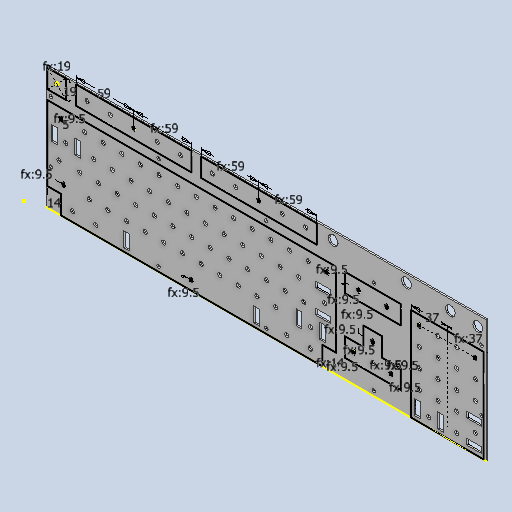
# Autodesk Inventor part: PCB
Saved by Autodesk Inventor 2025 (Build 290162000, 162)
## iProperties
Created: 2024-07-10
Part Number: PCB
Material: Generic
Document SubType Name: Modeling
Designer: adam
Density: 1 g/cm^3
Appearance: Default
Author: adam
Autodesk Inventor part; units mm, degrees
(part 1 of 2)
ref_plane "YZ Plane" through (0, 0, 0) normal (1, 0, 0) x (0, 1, 0)
ref_plane "XZ Plane" through (0, 0, 0) normal (0, 1, 0) x (-1, 0, 0)
ref_plane "XY Plane" through (0, 0, 0) normal (0, 0, 1) x (1, 0, 0)
sketch "Sketch2" plane through (0, 0, 0) normal (0, 0, 1) x (1, 0, 0)
  line L0 (313.1708, 72.3776) -> (298.1708, 72.3776) projected
  spline S0 degree 3 poles (439.2443, 124.4635) (438.3067, 125.4012) (437.0349, 125.928) (435.7088, 125.928) knots 0 0 0 0 1 1 1 1 projected
  line L1 (440.5, 108.25) -> (413, 108.25) projected
  spline S1 degree 3 poles (431.0894, 122.8414) (430.3155, 120.973) (430.7433, 118.8225) (432.1733, 117.3925) knots 0 0 0 0 1 1 1 1 projected
  spline S2 degree 3 poles (432.1733, 117.3925) (433.6033, 115.9625) (435.7538, 115.5347) (437.6222, 116.3086) knots 0 0 0 0 1 1 1 1 projected
  spline S3 degree 3 poles (435.7088, 125.928) (433.6865, 125.928) (431.8633, 124.7098) (431.0894, 122.8414) knots 0 0 0 0 1 1 1 1 projected
  line L2 (413, 115.25) -> (413, 127.25) projected
  line L3 (422.7108, 9.978) -> (422.7108, 24.978) projected
  line L4 (428.7108, 9.978) -> (422.7108, 9.978) projected
  line L5 (428.7108, 24.978) -> (428.7108, 9.978) projected
  line L6 (422.7108, 24.978) -> (428.7108, 24.978) projected
  line L7 (398.7108, 9.978) -> (398.7108, 24.978) projected
  line L8 (404.7108, 9.978) -> (398.7108, 9.978) projected
  line L9 (404.7108, 24.978) -> (404.7108, 9.978) projected
  line L10 (398.7108, 24.978) -> (404.7108, 24.978) projected
  line L11 (452.2088, 40.476) -> (452.2088, 34.476) projected
  spline S4 degree 3 poles (465.8832, 44.9197) (465.6123, 44.2658) (465.7621, 43.5131) (466.2626, 43.0126) knots 0 0 0 0 1 1 1 1 projected
  spline S5 degree 3 poles (467.5, 46) (466.7922, 46) (466.1541, 45.5736) (465.8832, 44.9197) knots 0 0 0 0 1 1 1 1 projected
  spline S6 degree 3 poles (466.2626, 43.0126) (466.7631, 42.5121) (467.5158, 42.3623) (468.1697, 42.6332) knots 0 0 0 0 1 1 1 1 projected
  spline S7 degree 3 poles (468.7374, 45.4874) (468.4092, 45.8156) (467.9641, 46) (467.5, 46) knots 0 0 0 0 1 1 1 1 projected
  spline S8 degree 3 poles (469.25, 44.25) (469.25, 44.7141) (469.0656, 45.1592) (468.7374, 45.4874) knots 0 0 0 0 1 1 1 1 projected
  spline S9 degree 3 poles (468.1697, 42.6332) (468.8236, 42.9041) (469.25, 43.5422) (469.25, 44.25) knots 0 0 0 0 1 1 1 1 projected
  spline S10 degree 3 poles (295.0681, 34.9296) (295.0681, 35.4922) (294.8446, 36.0318) (294.4468, 36.4296) knots 0 0 0 0 1 1 1 1 projected
  spline S11 degree 3 poles (358.7374, 107.6258) (358.4092, 107.954) (357.9641, 108.1384) (357.5, 108.1384) knots 0 0 0 0 1 1 1 1 projected
  spline S12 degree 3 poles (355.8832, 107.0581) (355.6123, 106.4042) (355.7621, 105.6515) (356.2626, 105.151) knots 0 0 0 0 1 1 1 1 projected
  spline S13 degree 3 poles (357.5, 108.1384) (356.7922, 108.1384) (356.1541, 107.712) (355.8832, 107.0581) knots 0 0 0 0 1 1 1 1 projected
  spline S14 degree 3 poles (356.2626, 105.151) (356.7631, 104.6505) (357.5158, 104.5007) (358.1697, 104.7716) knots 0 0 0 0 1 1 1 1 projected
  spline S15 degree 3 poles (358.1697, 104.7716) (358.8236, 105.0425) (359.25, 105.6806) (359.25, 106.3884) knots 0 0 0 0 1 1 1 1 projected
  line L12 (464, 108.25) -> (444.5, 108.25) projected
  spline S16 degree 3 poles (359.25, 106.3884) (359.25, 106.8525) (359.0656, 107.2976) (358.7374, 107.6258) knots 0 0 0 0 1 1 1 1 projected
  spline S17 degree 3 poles (440.7088, 120.928) (440.7088, 122.2541) (440.182, 123.5259) (439.2443, 124.4635) knots 0 0 0 0 1 1 1 1 projected
  spline S18 degree 3 poles (437.6222, 116.3086) (439.4906, 117.0825) (440.7088, 118.9057) (440.7088, 120.928) knots 0 0 0 0 1 1 1 1 projected
  spline S19 degree 3 poles (394.4023, 126.7719) (393.4647, 127.7096) (392.1929, 128.2364) (390.8668, 128.2364) knots 0 0 0 0 1 1 1 1 projected
  spline S20 degree 3 poles (395.8668, 123.2364) (395.8668, 124.5625) (395.34, 125.8343) (394.4023, 126.7719) knots 0 0 0 0 1 1 1 1 projected
  spline S21 degree 3 poles (392.7802, 118.617) (394.6486, 119.3909) (395.8668, 121.2141) (395.8668, 123.2364) knots 0 0 0 0 1 1 1 1 projected
  spline S22 degree 3 poles (387.3313, 119.7009) (388.7613, 118.2709) (390.9118, 117.8431) (392.7802, 118.617) knots 0 0 0 0 1 1 1 1 projected
  spline S23 degree 3 poles (386.2474, 125.1498) (385.4735, 123.2814) (385.9013, 121.1309) (387.3313, 119.7009) knots 0 0 0 0 1 1 1 1 projected
  spline S24 degree 3 poles (390.8668, 128.2364) (388.8445, 128.2364) (387.0213, 127.0182) (386.2474, 125.1498) knots 0 0 0 0 1 1 1 1 projected
  spline S25 degree 3 poles (465.8832, 107.0581) (465.6123, 106.4042) (465.7621, 105.6515) (466.2626, 105.151) knots 0 0 0 0 1 1 1 1 projected
  spline S26 degree 3 poles (466.2626, 105.151) (466.7631, 104.6505) (467.5158, 104.5007) (468.1697, 104.7716) knots 0 0 0 0 1 1 1 1 projected
  spline S27 degree 3 poles (467.5, 108.1384) (466.7922, 108.1384) (466.1541, 107.712) (465.8832, 107.0581) knots 0 0 0 0 1 1 1 1 projected
  spline S28 degree 3 poles (468.1697, 104.7716) (468.8236, 105.0425) (469.25, 105.6806) (469.25, 106.3884) knots 0 0 0 0 1 1 1 1 projected
  spline S29 degree 3 poles (468.7374, 107.6258) (468.4092, 107.954) (467.9641, 108.1384) (467.5, 108.1384) knots 0 0 0 0 1 1 1 1 projected
  spline S30 degree 3 poles (469.25, 106.3884) (469.25, 106.8525) (469.0656, 107.2976) (468.7374, 107.6258) knots 0 0 0 0 1 1 1 1 projected
  line L13 (413, 108.25) -> (413, 111.25) projected
  line L14 (452.2088, 16.476) -> (452.2088, 10.476) projected
  line L15 (467.2088, 16.476) -> (452.2088, 16.476) projected
  line L16 (467.2088, 10.476) -> (467.2088, 16.476) projected
  line L17 (452.2088, 10.476) -> (467.2088, 10.476) projected
  spline S31 degree 3 poles (467.2443, 124.4635) (466.3067, 125.4012) (465.0349, 125.928) (463.7088, 125.928) knots 0 0 0 0 1 1 1 1 projected
  line L18 (472.5, 131.25) -> (472.5, 6.25) projected
  spline S32 degree 3 poles (459.0894, 122.8414) (458.3155, 120.973) (458.7433, 118.8225) (460.1733, 117.3925) knots 0 0 0 0 1 1 1 1 projected
  spline S33 degree 3 poles (460.1733, 117.3925) (461.6033, 115.9625) (463.7538, 115.5347) (465.6222, 116.3086) knots 0 0 0 0 1 1 1 1 projected
  spline S34 degree 3 poles (463.7088, 125.928) (461.6865, 125.928) (459.8633, 124.7098) (459.0894, 122.8414) knots 0 0 0 0 1 1 1 1 projected
  spline S35 degree 3 poles (465.6222, 116.3086) (467.4906, 117.0825) (468.7088, 118.9057) (468.7088, 120.928) knots 0 0 0 0 1 1 1 1 projected
  spline S36 degree 3 poles (468.7088, 120.928) (468.7088, 122.2541) (468.182, 123.5259) (467.2443, 124.4635) knots 0 0 0 0 1 1 1 1 projected
  spline S37 degree 3 poles (206.0548, 74.5296) (205.657, 74.9274) (205.1174, 75.1509) (204.5548, 75.1509) knots 0 0 0 0 1 1 1 1 projected
  spline S38 degree 3 poles (206.6761, 73.0296) (206.6761, 73.5922) (206.4526, 74.1318) (206.0548, 74.5296) knots 0 0 0 0 1 1 1 1 projected
  spline S39 degree 3 poles (205.3666, 71.0698) (206.1593, 71.3981) (206.6761, 72.1716) (206.6761, 73.0296) knots 0 0 0 0 1 1 1 1 projected
  spline S40 degree 3 poles (203.0548, 71.5296) (203.6615, 70.9229) (204.5739, 70.7414) (205.3666, 71.0698) knots 0 0 0 0 1 1 1 1 projected
  spline S41 degree 3 poles (202.595, 73.8414) (202.2666, 73.0487) (202.4481, 72.1363) (203.0548, 71.5296) knots 0 0 0 0 1 1 1 1 projected
  spline S42 degree 3 poles (204.5548, 75.1509) (203.6968, 75.1509) (202.9233, 74.6341) (202.595, 73.8414) knots 0 0 0 0 1 1 1 1 projected
  spline S43 degree 3 poles (167.9548, 74.5296) (167.557, 74.9274) (167.0174, 75.1509) (166.4548, 75.1509) knots 0 0 0 0 1 1 1 1 projected
  spline S44 degree 3 poles (168.5761, 73.0296) (168.5761, 73.5922) (168.3526, 74.1318) (167.9548, 74.5296) knots 0 0 0 0 1 1 1 1 projected
  spline S45 degree 3 poles (167.2666, 71.0698) (168.0593, 71.3981) (168.5761, 72.1716) (168.5761, 73.0296) knots 0 0 0 0 1 1 1 1 projected
  spline S46 degree 3 poles (164.9548, 71.5296) (165.5615, 70.9229) (166.4739, 70.7414) (167.2666, 71.0698) knots 0 0 0 0 1 1 1 1 projected
  spline S47 degree 3 poles (164.495, 73.8414) (164.1666, 73.0487) (164.3481, 72.1363) (164.9548, 71.5296) knots 0 0 0 0 1 1 1 1 projected
  spline S48 degree 3 poles (166.4548, 75.1509) (165.5968, 75.1509) (164.8233, 74.6341) (164.495, 73.8414) knots 0 0 0 0 1 1 1 1 projected
  spline S49 degree 3 poles (187.0048, 74.5296) (186.607, 74.9274) (186.0674, 75.1509) (185.5048, 75.1509) knots 0 0 0 0 1 1 1 1 projected
  spline S50 degree 3 poles (183.545, 73.8414) (183.2166, 73.0487) (183.3981, 72.1363) (184.0048, 71.5296) knots 0 0 0 0 1 1 1 1 projected
  spline S51 degree 3 poles (187.6261, 73.0296) (187.6261, 73.5922) (187.4026, 74.1318) (187.0048, 74.5296) knots 0 0 0 0 1 1 1 1 projected
  spline S52 degree 3 poles (184.0048, 71.5296) (184.6115, 70.9229) (185.5239, 70.7414) (186.3166, 71.0698) knots 0 0 0 0 1 1 1 1 projected
  spline S53 degree 3 poles (186.3166, 71.0698) (187.1093, 71.3981) (187.6261, 72.1716) (187.6261, 73.0296) knots 0 0 0 0 1 1 1 1 projected
  spline S54 degree 3 poles (185.5048, 75.1509) (184.6468, 75.1509) (183.8733, 74.6341) (183.545, 73.8414) knots 0 0 0 0 1 1 1 1 projected
  spline S55 degree 3 poles (172.2728, 17.3796) (171.875, 17.7774) (171.3354, 18.0009) (170.7728, 18.0009) knots 0 0 0 0 1 1 1 1 projected
  spline S56 degree 3 poles (172.8941, 15.8796) (172.8941, 16.4422) (172.6706, 16.9818) (172.2728, 17.3796) knots 0 0 0 0 1 1 1 1 projected
  spline S57 degree 3 poles (171.5846, 13.9198) (172.3773, 14.2481) (172.8941, 15.0216) (172.8941, 15.8796) knots 0 0 0 0 1 1 1 1 projected
  spline S58 degree 3 poles (169.2728, 14.3796) (169.8795, 13.7729) (170.7919, 13.5914) (171.5846, 13.9198) knots 0 0 0 0 1 1 1 1 projected
  spline S59 degree 3 poles (168.813, 16.6914) (168.4846, 15.8987) (168.6661, 14.9863) (169.2728, 14.3796) knots 0 0 0 0 1 1 1 1 projected
  spline S60 degree 3 poles (170.7728, 18.0009) (169.9148, 18.0009) (169.1413, 17.4841) (168.813, 16.6914) knots 0 0 0 0 1 1 1 1 projected
  spline S61 degree 3 poles (201.4828, 36.4296) (201.085, 36.8274) (200.5454, 37.0509) (199.9828, 37.0509) knots 0 0 0 0 1 1 1 1 projected
  spline S62 degree 3 poles (202.1041, 34.9296) (202.1041, 35.4922) (201.8806, 36.0318) (201.4828, 36.4296) knots 0 0 0 0 1 1 1 1 projected
  spline S63 degree 3 poles (200.7946, 32.9698) (201.5873, 33.2981) (202.1041, 34.0716) (202.1041, 34.9296) knots 0 0 0 0 1 1 1 1 projected
  spline S64 degree 3 poles (198.4828, 33.4296) (199.0895, 32.8229) (200.0019, 32.6414) (200.7946, 32.9698) knots 0 0 0 0 1 1 1 1 projected
  spline S65 degree 3 poles (198.023, 35.7414) (197.6946, 34.9487) (197.8761, 34.0363) (198.4828, 33.4296) knots 0 0 0 0 1 1 1 1 projected
  spline S66 degree 3 poles (199.9828, 37.0509) (199.1248, 37.0509) (198.3513, 36.5341) (198.023, 35.7414) knots 0 0 0 0 1 1 1 1 projected
  spline S67 degree 3 poles (169.321, 54.7914) (168.9926, 53.9987) (169.1741, 53.0863) (169.7808, 52.4796) knots 0 0 0 0 1 1 1 1 projected
  spline S68 degree 3 poles (171.2808, 56.1009) (170.4228, 56.1009) (169.6493, 55.5841) (169.321, 54.7914) knots 0 0 0 0 1 1 1 1 projected
  spline S69 degree 3 poles (169.7808, 52.4796) (170.3875, 51.8729) (171.2999, 51.6914) (172.0926, 52.0198) knots 0 0 0 0 1 1 1 1 projected
  spline S70 degree 3 poles (172.7808, 55.4796) (172.383, 55.8774) (171.8434, 56.1009) (171.2808, 56.1009) knots 0 0 0 0 1 1 1 1 projected
  spline S71 degree 3 poles (172.0926, 52.0198) (172.8853, 52.3481) (173.4021, 53.1216) (173.4021, 53.9796) knots 0 0 0 0 1 1 1 1 projected
  spline S72 degree 3 poles (178.973, 35.7414) (178.6446, 34.9487) (178.8261, 34.0363) (179.4328, 33.4296) knots 0 0 0 0 1 1 1 1 projected
  spline S73 degree 3 poles (180.9328, 37.0509) (180.0748, 37.0509) (179.3013, 36.5341) (178.973, 35.7414) knots 0 0 0 0 1 1 1 1 projected
  spline S74 degree 3 poles (179.4328, 33.4296) (180.0395, 32.8229) (180.9519, 32.6414) (181.7446, 32.9698) knots 0 0 0 0 1 1 1 1 projected
  spline S75 degree 3 poles (182.4328, 36.4296) (182.035, 36.8274) (181.4954, 37.0509) (180.9328, 37.0509) knots 0 0 0 0 1 1 1 1 projected
  spline S76 degree 3 poles (181.7446, 32.9698) (182.5373, 33.2981) (183.0541, 34.0716) (183.0541, 34.9296) knots 0 0 0 0 1 1 1 1 projected
  spline S77 degree 3 poles (183.0541, 34.9296) (183.0541, 35.4922) (182.8306, 36.0318) (182.4328, 36.4296) knots 0 0 0 0 1 1 1 1 projected
  spline S78 degree 3 poles (188.371, 54.7914) (188.0426, 53.9987) (188.2241, 53.0863) (188.8308, 52.4796) knots 0 0 0 0 1 1 1 1 projected
  spline S79 degree 3 poles (190.3308, 56.1009) (189.4728, 56.1009) (188.6993, 55.5841) (188.371, 54.7914) knots 0 0 0 0 1 1 1 1 projected
  spline S80 degree 3 poles (188.8308, 52.4796) (189.4375, 51.8729) (190.3499, 51.6914) (191.1426, 52.0198) knots 0 0 0 0 1 1 1 1 projected
  spline S81 degree 3 poles (191.8308, 55.4796) (191.433, 55.8774) (190.8934, 56.1009) (190.3308, 56.1009) knots 0 0 0 0 1 1 1 1 projected
  spline S82 degree 3 poles (191.1426, 52.0198) (191.9353, 52.3481) (192.4521, 53.1216) (192.4521, 53.9796) knots 0 0 0 0 1 1 1 1 projected
  spline S83 degree 3 poles (192.4521, 53.9796) (192.4521, 54.5422) (192.2286, 55.0818) (191.8308, 55.4796) knots 0 0 0 0 1 1 1 1 projected
  spline S84 degree 3 poles (173.4021, 53.9796) (173.4021, 54.5422) (173.1786, 55.0818) (172.7808, 55.4796) knots 0 0 0 0 1 1 1 1 projected
  spline S85 degree 3 poles (159.1781, 92.0796) (159.1781, 93.2512) (158.2284, 94.2009) (157.0568, 94.2009) knots 0 0 0 0 1 1 1 1 projected
  spline S86 degree 3 poles (157.8686, 90.1198) (158.6613, 90.4481) (159.1781, 91.2216) (159.1781, 92.0796) knots 0 0 0 0 1 1 1 1 projected
  spline S87 degree 3 poles (193.6568, 90.5796) (194.2635, 89.9729) (195.1759, 89.7914) (195.9686, 90.1198) knots 0 0 0 0 1 1 1 1 projected
  spline S88 degree 3 poles (174.6068, 90.5796) (175.2135, 89.9729) (176.1259, 89.7914) (176.9186, 90.1198) knots 0 0 0 0 1 1 1 1 projected
  spline S89 degree 3 poles (176.9186, 90.1198) (177.7113, 90.4481) (178.2281, 91.2216) (178.2281, 92.0796) knots 0 0 0 0 1 1 1 1 projected
  spline S90 degree 3 poles (193.197, 92.8914) (192.8686, 92.0987) (193.0501, 91.1863) (193.6568, 90.5796) knots 0 0 0 0 1 1 1 1 projected
  spline S91 degree 3 poles (195.9686, 90.1198) (196.7613, 90.4481) (197.2781, 91.2216) (197.2781, 92.0796) knots 0 0 0 0 1 1 1 1 projected
  spline S92 degree 3 poles (197.2781, 92.0796) (197.2781, 92.6422) (197.0546, 93.1818) (196.6568, 93.5796) knots 0 0 0 0 1 1 1 1 projected
  spline S93 degree 3 poles (196.6568, 93.5796) (196.259, 93.9774) (195.7194, 94.2009) (195.1568, 94.2009) knots 0 0 0 0 1 1 1 1 projected
  spline S94 degree 3 poles (178.2281, 92.0796) (178.2281, 92.6422) (178.0046, 93.1818) (177.6068, 93.5796) knots 0 0 0 0 1 1 1 1 projected
  spline S95 degree 3 poles (195.1568, 94.2009) (194.2988, 94.2009) (193.5253, 93.6841) (193.197, 92.8914) knots 0 0 0 0 1 1 1 1 projected
  spline S96 degree 3 poles (177.6068, 93.5796) (177.209, 93.9774) (176.6694, 94.2009) (176.1068, 94.2009) knots 0 0 0 0 1 1 1 1 projected
  spline S97 degree 3 poles (176.1068, 94.2009) (175.2488, 94.2009) (174.4753, 93.6841) (174.147, 92.8914) knots 0 0 0 0 1 1 1 1 projected
  spline S98 degree 3 poles (155.5568, 90.5796) (156.1635, 89.9729) (157.0759, 89.7914) (157.8686, 90.1198) knots 0 0 0 0 1 1 1 1 projected
  spline S99 degree 3 poles (155.097, 92.8914) (154.7686, 92.0987) (154.9501, 91.1863) (155.5568, 90.5796) knots 0 0 0 0 1 1 1 1 projected
  spline S100 degree 3 poles (157.0568, 94.2009) (156.1988, 94.2009) (155.4253, 93.6841) (155.097, 92.8914) knots 0 0 0 0 1 1 1 1 projected
  spline S101 degree 3 poles (190.8568, 119.2364) (191.4635, 118.6297) (192.3759, 118.4482) (193.1686, 118.7766) knots 0 0 0 0 1 1 1 1 projected
  spline S102 degree 3 poles (193.1686, 118.7766) (193.9613, 119.1049) (194.4781, 119.8784) (194.4781, 120.7364) knots 0 0 0 0 1 1 1 1 projected
  spline S103 degree 3 poles (190.397, 121.5482) (190.0686, 120.7555) (190.2501, 119.8431) (190.8568, 119.2364) knots 0 0 0 0 1 1 1 1 projected
  spline S104 degree 3 poles (194.4781, 120.7364) (194.4781, 121.299) (194.2546, 121.8386) (193.8568, 122.2364) knots 0 0 0 0 1 1 1 1 projected
  spline S105 degree 3 poles (193.8568, 122.2364) (193.459, 122.6342) (192.9194, 122.8577) (192.3568, 122.8577) knots 0 0 0 0 1 1 1 1 projected
  spline S106 degree 3 poles (192.3568, 122.8577) (191.4988, 122.8577) (190.7253, 122.3409) (190.397, 121.5482) knots 0 0 0 0 1 1 1 1 projected
  spline S107 degree 3 poles (158.3508, 119.2364) (158.9575, 118.6297) (159.8699, 118.4482) (160.6626, 118.7766) knots 0 0 0 0 1 1 1 1 projected
  spline S108 degree 3 poles (160.6626, 118.7766) (161.4553, 119.1049) (161.9721, 119.8784) (161.9721, 120.7364) knots 0 0 0 0 1 1 1 1 projected
  spline S109 degree 3 poles (161.9721, 120.7364) (161.9721, 121.299) (161.7486, 121.8386) (161.3508, 122.2364) knots 0 0 0 0 1 1 1 1 projected
  spline S110 degree 3 poles (157.891, 121.5482) (157.5626, 120.7555) (157.7441, 119.8431) (158.3508, 119.2364) knots 0 0 0 0 1 1 1 1 projected
  spline S111 degree 3 poles (161.3508, 122.2364) (160.953, 122.6342) (160.4134, 122.8577) (159.8508, 122.8577) knots 0 0 0 0 1 1 1 1 projected
  spline S112 degree 3 poles (159.8508, 122.8577) (158.9928, 122.8577) (158.2193, 122.3409) (157.891, 121.5482) knots 0 0 0 0 1 1 1 1 projected
  spline S113 degree 3 poles (174.147, 92.8914) (173.8186, 92.0987) (174.0001, 91.1863) (174.6068, 90.5796) knots 0 0 0 0 1 1 1 1 projected
  spline S114 degree 3 poles (164.0041, 34.9296) (164.0041, 36.1012) (163.0544, 37.0509) (161.8828, 37.0509) knots 0 0 0 0 1 1 1 1 projected
  spline S115 degree 3 poles (162.6946, 32.9698) (163.4873, 33.2981) (164.0041, 34.0716) (164.0041, 34.9296) knots 0 0 0 0 1 1 1 1 projected
  spline S116 degree 3 poles (160.3828, 33.4296) (160.9895, 32.8229) (161.9019, 32.6414) (162.6946, 32.9698) knots 0 0 0 0 1 1 1 1 projected
  spline S117 degree 3 poles (159.923, 35.7414) (159.5946, 34.9487) (159.7761, 34.0363) (160.3828, 33.4296) knots 0 0 0 0 1 1 1 1 projected
  spline S118 degree 3 poles (161.8828, 37.0509) (161.0248, 37.0509) (160.2513, 36.5341) (159.923, 35.7414) knots 0 0 0 0 1 1 1 1 projected
  spline S119 degree 3 poles (154.3521, 53.9796) (154.3521, 55.1512) (153.4024, 56.1009) (152.2308, 56.1009) knots 0 0 0 0 1 1 1 1 projected
  spline S120 degree 3 poles (153.0426, 52.0198) (153.8353, 52.3481) (154.3521, 53.1216) (154.3521, 53.9796) knots 0 0 0 0 1 1 1 1 projected
  spline S121 degree 3 poles (150.271, 54.7914) (149.9426, 53.9987) (150.1241, 53.0863) (150.7308, 52.4796) knots 0 0 0 0 1 1 1 1 projected
  spline S122 degree 3 poles (150.7308, 52.4796) (151.3375, 51.8729) (152.2499, 51.6914) (153.0426, 52.0198) knots 0 0 0 0 1 1 1 1 projected
  spline S123 degree 3 poles (152.2308, 56.1009) (151.3728, 56.1009) (150.5993, 55.5841) (150.271, 54.7914) knots 0 0 0 0 1 1 1 1 projected
  spline S124 degree 3 poles (139.25, 11.25) (139.25, 11.7141) (139.0656, 12.1592) (138.7374, 12.4874) knots 0 0 0 0 1 1 1 1 projected
  spline S125 degree 3 poles (138.7374, 12.4874) (138.4092, 12.8156) (137.9641, 13) (137.5, 13) knots 0 0 0 0 1 1 1 1 projected
  spline S126 degree 3 poles (138.1697, 9.6332) (138.8236, 9.9041) (139.25, 10.5422) (139.25, 11.25) knots 0 0 0 0 1 1 1 1 projected
  spline S127 degree 3 poles (137.5, 13) (136.7922, 13) (136.1541, 12.5736) (135.8832, 11.9197) knots 0 0 0 0 1 1 1 1 projected
  spline S128 degree 3 poles (135.8832, 11.9197) (135.6123, 11.2658) (135.7621, 10.5131) (136.2626, 10.0126) knots 0 0 0 0 1 1 1 1 projected
  spline S129 degree 3 poles (136.2626, 10.0126) (136.7631, 9.5121) (137.5158, 9.3623) (138.1697, 9.6332) knots 0 0 0 0 1 1 1 1 projected
  spline S130 degree 3 poles (148.9048, 74.4508) (148.507, 74.8486) (147.9674, 75.0721) (147.4048, 75.0721) knots 0 0 0 0 1 1 1 1 projected
  spline S131 degree 3 poles (149.5261, 72.9508) (149.5261, 73.5134) (149.3026, 74.053) (148.9048, 74.4508) knots 0 0 0 0 1 1 1 1 projected
  spline S132 degree 3 poles (120.4568, 93.5796) (120.059, 93.9774) (119.5194, 94.2009) (118.9568, 94.2009) knots 0 0 0 0 1 1 1 1 projected
  spline S133 degree 3 poles (118.9568, 94.2009) (117.7852, 94.2009) (116.8355, 93.2512) (116.8355, 92.0796) knots 0 0 0 0 1 1 1 1 projected
  spline S134 degree 3 poles (121.0781, 92.0796) (121.0781, 92.6422) (120.8546, 93.1818) (120.4568, 93.5796) knots 0 0 0 0 1 1 1 1 projected
  spline S135 degree 3 poles (116.8355, 92.0796) (116.8355, 90.908) (117.7852, 89.9583) (118.9568, 89.9583) knots 0 0 0 0 1 1 1 1 projected
  spline S136 degree 3 poles (118.9568, 89.9583) (120.1284, 89.9583) (121.0781, 90.908) (121.0781, 92.0796) knots 0 0 0 0 1 1 1 1 projected
  spline S137 degree 3 poles (138.0068, 94.2009) (137.1488, 94.2009) (136.3753, 93.6841) (136.047, 92.8914) knots 0 0 0 0 1 1 1 1 projected
  spline S138 degree 3 poles (139.5068, 93.5796) (139.109, 93.9774) (138.5694, 94.2009) (138.0068, 94.2009) knots 0 0 0 0 1 1 1 1 projected
  spline S139 degree 3 poles (140.1281, 92.0796) (140.1281, 92.6422) (139.9046, 93.1818) (139.5068, 93.5796) knots 0 0 0 0 1 1 1 1 projected
  spline S140 degree 3 poles (136.047, 92.8914) (135.7186, 92.0987) (135.9001, 91.1863) (136.5068, 90.5796) knots 0 0 0 0 1 1 1 1 projected
  spline S141 degree 3 poles (138.8186, 90.1198) (139.6113, 90.4481) (140.1281, 91.2216) (140.1281, 92.0796) knots 0 0 0 0 1 1 1 1 projected
  spline S142 degree 3 poles (129.8548, 74.5296) (129.457, 74.9274) (128.9174, 75.1509) (128.3548, 75.1509) knots 0 0 0 0 1 1 1 1 projected
  spline S143 degree 3 poles (147.4048, 75.0721) (146.5468, 75.0721) (145.7733, 74.5553) (145.445, 73.7626) knots 0 0 0 0 1 1 1 1 projected
  spline S144 degree 3 poles (145.445, 73.7626) (145.1166, 72.9699) (145.2981, 72.0575) (145.9048, 71.4508) knots 0 0 0 0 1 1 1 1 projected
  spline S145 degree 3 poles (148.2166, 70.991) (149.0093, 71.3193) (149.5261, 72.0928) (149.5261, 72.9508) knots 0 0 0 0 1 1 1 1 projected
  spline S146 degree 3 poles (145.9048, 71.4508) (146.5115, 70.8441) (147.4239, 70.6626) (148.2166, 70.991) knots 0 0 0 0 1 1 1 1 projected
  spline S147 degree 3 poles (128.3548, 75.1509) (127.4968, 75.1509) (126.7233, 74.6341) (126.395, 73.8414) knots 0 0 0 0 1 1 1 1 projected
  spline S148 degree 3 poles (130.4761, 73.0296) (130.4761, 73.5922) (130.2526, 74.1318) (129.8548, 74.5296) knots 0 0 0 0 1 1 1 1 projected
  spline S149 degree 3 poles (126.395, 73.8414) (126.0666, 73.0487) (126.2481, 72.1363) (126.8548, 71.5296) knots 0 0 0 0 1 1 1 1 projected
  spline S150 degree 3 poles (129.1666, 71.0698) (129.9593, 71.3981) (130.4761, 72.1716) (130.4761, 73.0296) knots 0 0 0 0 1 1 1 1 projected
  spline S151 degree 3 poles (126.8548, 71.5296) (127.4615, 70.9229) (128.3739, 70.7414) (129.1666, 71.0698) knots 0 0 0 0 1 1 1 1 projected
  spline S152 degree 3 poles (136.5068, 90.5796) (137.1135, 89.9729) (138.0259, 89.7914) (138.8186, 90.1198) knots 0 0 0 0 1 1 1 1 projected
  spline S153 degree 3 poles (138.7374, 107.6258) (138.4092, 107.954) (137.9641, 108.1384) (137.5, 108.1384) knots 0 0 0 0 1 1 1 1 projected
  spline S154 degree 3 poles (139.25, 106.3884) (139.25, 106.8525) (139.0656, 107.2976) (138.7374, 107.6258) knots 0 0 0 0 1 1 1 1 projected
  spline S155 degree 3 poles (138.1697, 104.7716) (138.8236, 105.0425) (139.25, 105.6806) (139.25, 106.3884) knots 0 0 0 0 1 1 1 1 projected
  spline S156 degree 3 poles (136.2626, 105.151) (136.7631, 104.6505) (137.5158, 104.5007) (138.1697, 104.7716) knots 0 0 0 0 1 1 1 1 projected
  spline S157 degree 3 poles (135.8832, 107.0581) (135.6123, 106.4042) (135.7621, 105.6515) (136.2626, 105.151) knots 0 0 0 0 1 1 1 1 projected
  spline S158 degree 3 poles (137.5, 108.1384) (136.7922, 108.1384) (136.1541, 107.712) (135.8832, 107.0581) knots 0 0 0 0 1 1 1 1 projected
  spline S159 degree 3 poles (134.4748, 119.2364) (135.0815, 118.6297) (135.9939, 118.4482) (136.7866, 118.7766) knots 0 0 0 0 1 1 1 1 projected
  spline S160 degree 3 poles (136.7866, 118.7766) (137.5793, 119.1049) (138.0961, 119.8784) (138.0961, 120.7364) knots 0 0 0 0 1 1 1 1 projected
  spline S161 degree 3 poles (134.015, 121.5482) (133.6866, 120.7555) (133.8681, 119.8431) (134.4748, 119.2364) knots 0 0 0 0 1 1 1 1 projected
  spline S162 degree 3 poles (137.4748, 122.2364) (137.077, 122.6342) (136.5374, 122.8577) (135.9748, 122.8577) knots 0 0 0 0 1 1 1 1 projected
  spline S163 degree 3 poles (135.9748, 122.8577) (135.1168, 122.8577) (134.3433, 122.3409) (134.015, 121.5482) knots 0 0 0 0 1 1 1 1 projected
  spline S164 degree 3 poles (112.9106, 118.7486) (113.7033, 119.0769) (114.2201, 119.8504) (114.2201, 120.7084) knots 0 0 0 0 1 1 1 1 projected
  spline S165 degree 3 poles (110.5988, 119.2084) (111.2055, 118.6017) (112.1179, 118.4202) (112.9106, 118.7486) knots 0 0 0 0 1 1 1 1 projected
  spline S166 degree 3 poles (114.2201, 120.7084) (114.2201, 121.271) (113.9966, 121.8106) (113.5988, 122.2084) knots 0 0 0 0 1 1 1 1 projected
  spline S167 degree 3 poles (113.5988, 122.2084) (113.201, 122.6062) (112.6614, 122.8297) (112.0988, 122.8297) knots 0 0 0 0 1 1 1 1 projected
  spline S168 degree 3 poles (110.139, 121.5202) (109.8106, 120.7275) (109.9921, 119.8151) (110.5988, 119.2084) knots 0 0 0 0 1 1 1 1 projected
  spline S169 degree 3 poles (112.0988, 122.8297) (111.2408, 122.8297) (110.4673, 122.3129) (110.139, 121.5202) knots 0 0 0 0 1 1 1 1 projected
  spline S170 degree 3 poles (138.0961, 120.7364) (138.0961, 121.299) (137.8726, 121.8386) (137.4748, 122.2364) knots 0 0 0 0 1 1 1 1 projected
  line L19 (101.6246, 24.8046) -> (107.6246, 24.8046) projected
  spline S171 degree 3 poles (135.3021, 53.9796) (135.3021, 54.5422) (135.0786, 55.0818) (134.6808, 55.4796) knots 0 0 0 0 1 1 1 1 projected
  spline S172 degree 3 poles (133.9926, 52.0198) (134.7853, 52.3481) (135.3021, 53.1216) (135.3021, 53.9796) knots 0 0 0 0 1 1 1 1 projected
  spline S173 degree 3 poles (134.6808, 55.4796) (134.283, 55.8774) (133.7434, 56.1009) (133.1808, 56.1009) knots 0 0 0 0 1 1 1 1 projected
  spline S174 degree 3 poles (131.6808, 52.4796) (132.2875, 51.8729) (133.1999, 51.6914) (133.9926, 52.0198) knots 0 0 0 0 1 1 1 1 projected
  spline S175 degree 3 poles (144.3328, 36.4296) (143.935, 36.8274) (143.3954, 37.0509) (142.8328, 37.0509) knots 0 0 0 0 1 1 1 1 projected
  spline S176 degree 3 poles (133.1808, 56.1009) (132.3228, 56.1009) (131.5493, 55.5841) (131.221, 54.7914) knots 0 0 0 0 1 1 1 1 projected
  spline S177 degree 3 poles (131.221, 54.7914) (130.8926, 53.9987) (131.0741, 53.0863) (131.6808, 52.4796) knots 0 0 0 0 1 1 1 1 projected
  spline S178 degree 3 poles (144.9541, 34.9296) (144.9541, 35.4922) (144.7306, 36.0318) (144.3328, 36.4296) knots 0 0 0 0 1 1 1 1 projected
  spline S179 degree 3 poles (142.8328, 37.0509) (141.9748, 37.0509) (141.2013, 36.5341) (140.873, 35.7414) knots 0 0 0 0 1 1 1 1 projected
  spline S180 degree 3 poles (140.873, 35.7414) (140.5446, 34.9487) (140.7261, 34.0363) (141.3328, 33.4296) knots 0 0 0 0 1 1 1 1 projected
  spline S181 degree 3 poles (141.3328, 33.4296) (141.9395, 32.8229) (142.8519, 32.6414) (143.6446, 32.9698) knots 0 0 0 0 1 1 1 1 projected
  spline S182 degree 3 poles (125.9041, 34.9296) (125.9041, 35.4922) (125.6806, 36.0318) (125.2828, 36.4296) knots 0 0 0 0 1 1 1 1 projected
  spline S183 degree 3 poles (125.2828, 36.4296) (124.885, 36.8274) (124.3454, 37.0509) (123.7828, 37.0509) knots 0 0 0 0 1 1 1 1 projected
  spline S184 degree 3 poles (116.2521, 53.9796) (116.2521, 54.5422) (116.0286, 55.0818) (115.6308, 55.4796) knots 0 0 0 0 1 1 1 1 projected
  spline S185 degree 3 poles (114.9426, 52.0198) (115.7353, 52.3481) (116.2521, 53.1216) (116.2521, 53.9796) knots 0 0 0 0 1 1 1 1 projected
  spline S186 degree 3 poles (115.6308, 55.4796) (115.233, 55.8774) (114.6934, 56.1009) (114.1308, 56.1009) knots 0 0 0 0 1 1 1 1 projected
  spline S187 degree 3 poles (114.1308, 56.1009) (113.2728, 56.1009) (112.4993, 55.5841) (112.171, 54.7914) knots 0 0 0 0 1 1 1 1 projected
  spline S188 degree 3 poles (112.171, 54.7914) (111.8426, 53.9987) (112.0241, 53.0863) (112.6308, 52.4796) knots 0 0 0 0 1 1 1 1 projected
  spline S189 degree 3 poles (112.6308, 52.4796) (113.2375, 51.8729) (114.1499, 51.6914) (114.9426, 52.0198) knots 0 0 0 0 1 1 1 1 projected
  spline S190 degree 3 poles (124.5946, 32.9698) (125.3873, 33.2981) (125.9041, 34.0716) (125.9041, 34.9296) knots 0 0 0 0 1 1 1 1 projected
  spline S191 degree 3 poles (123.7828, 37.0509) (122.9248, 37.0509) (122.1513, 36.5341) (121.823, 35.7414) knots 0 0 0 0 1 1 1 1 projected
  spline S192 degree 3 poles (122.2828, 33.4296) (122.8895, 32.8229) (123.8019, 32.6414) (124.5946, 32.9698) knots 0 0 0 0 1 1 1 1 projected
  spline S193 degree 3 poles (121.823, 35.7414) (121.4946, 34.9487) (121.6761, 34.0363) (122.2828, 33.4296) knots 0 0 0 0 1 1 1 1 projected
  spline S194 degree 3 poles (106.8541, 34.9296) (106.8541, 35.4922) (106.6306, 36.0318) (106.2328, 36.4296) knots 0 0 0 0 1 1 1 1 projected
  spline S195 degree 3 poles (106.2328, 36.4296) (105.835, 36.8274) (105.2954, 37.0509) (104.7328, 37.0509) knots 0 0 0 0 1 1 1 1 projected
  spline S196 degree 3 poles (105.5446, 32.9698) (106.3373, 33.2981) (106.8541, 34.0716) (106.8541, 34.9296) knots 0 0 0 0 1 1 1 1 projected
  spline S197 degree 3 poles (104.7328, 37.0509) (103.8748, 37.0509) (103.1013, 36.5341) (102.773, 35.7414) knots 0 0 0 0 1 1 1 1 projected
  spline S198 degree 3 poles (102.773, 35.7414) (102.4446, 34.9487) (102.6261, 34.0363) (103.2328, 33.4296) knots 0 0 0 0 1 1 1 1 projected
  spline S199 degree 3 poles (103.2328, 33.4296) (103.8395, 32.8229) (104.7519, 32.6414) (105.5446, 32.9698) knots 0 0 0 0 1 1 1 1 projected
  spline S200 degree 3 poles (143.6446, 32.9698) (144.4373, 33.2981) (144.9541, 34.0716) (144.9541, 34.9296) knots 0 0 0 0 1 1 1 1 projected
  spline S201 degree 3 poles (111.4261, 73.0296) (111.4261, 73.5922) (111.2026, 74.1318) (110.8048, 74.5296) knots 0 0 0 0 1 1 1 1 projected
  spline S202 degree 3 poles (110.8048, 74.5296) (110.407, 74.9274) (109.8674, 75.1509) (109.3048, 75.1509) knots 0 0 0 0 1 1 1 1 projected
  spline S203 degree 3 poles (110.1166, 71.0698) (110.9093, 71.3981) (111.4261, 72.1716) (111.4261, 73.0296) knots 0 0 0 0 1 1 1 1 projected
  spline S204 degree 3 poles (109.3048, 75.1509) (108.4468, 75.1509) (107.6733, 74.6341) (107.345, 73.8414) knots 0 0 0 0 1 1 1 1 projected
  spline S205 degree 3 poles (107.8048, 71.5296) (108.4115, 70.9229) (109.3239, 70.7414) (110.1166, 71.0698) knots 0 0 0 0 1 1 1 1 projected
  spline S206 degree 3 poles (107.345, 73.8414) (107.0166, 73.0487) (107.1981, 72.1363) (107.8048, 71.5296) knots 0 0 0 0 1 1 1 1 projected
  spline S207 degree 3 poles (102.0281, 92.0796) (102.0281, 92.6422) (101.8046, 93.1818) (101.4068, 93.5796) knots 0 0 0 0 1 1 1 1 projected
  spline S208 degree 3 poles (100.7186, 90.1198) (101.5113, 90.4481) (102.0281, 91.2216) (102.0281, 92.0796) knots 0 0 0 0 1 1 1 1 projected
  spline S209 degree 3 poles (101.4068, 93.5796) (101.009, 93.9774) (100.4694, 94.2009) (99.9068, 94.2009) knots 0 0 0 0 1 1 1 1 projected
  spline S210 degree 3 poles (99.9068, 94.2009) (99.0488, 94.2009) (98.2753, 93.6841) (97.947, 92.8914) knots 0 0 0 0 1 1 1 1 projected
  spline S211 degree 3 poles (98.4068, 90.5796) (99.0135, 89.9729) (99.9259, 89.7914) (100.7186, 90.1198) knots 0 0 0 0 1 1 1 1 projected
  spline S212 degree 3 poles (92.3761, 73.0296) (92.3761, 73.5922) (92.1526, 74.1318) (91.7548, 74.5296) knots 0 0 0 0 1 1 1 1 projected
  spline S213 degree 3 poles (91.7548, 74.5296) (91.357, 74.9274) (90.8174, 75.1509) (90.2548, 75.1509) knots 0 0 0 0 1 1 1 1 projected
  spline S214 degree 3 poles (91.0666, 71.0698) (91.8593, 71.3981) (92.3761, 72.1716) (92.3761, 73.0296) knots 0 0 0 0 1 1 1 1 projected
  spline S215 degree 3 poles (90.2548, 75.1509) (89.3968, 75.1509) (88.6233, 74.6341) (88.295, 73.8414) knots 0 0 0 0 1 1 1 1 projected
  spline S216 degree 3 poles (88.7548, 71.5296) (89.3615, 70.9229) (90.2739, 70.7414) (91.0666, 71.0698) knots 0 0 0 0 1 1 1 1 projected
  spline S217 degree 3 poles (88.295, 73.8414) (87.9666, 73.0487) (88.1481, 72.1363) (88.7548, 71.5296) knots 0 0 0 0 1 1 1 1 projected
  spline S218 degree 3 poles (97.947, 92.8914) (97.6186, 92.0987) (97.8001, 91.1863) (98.4068, 90.5796) knots 0 0 0 0 1 1 1 1 projected
  spline S219 degree 3 poles (89.0346, 118.7766) (89.8273, 119.1049) (90.3441, 119.8784) (90.3441, 120.7364) knots 0 0 0 0 1 1 1 1 projected
  spline S220 degree 3 poles (72.7048, 74.5296) (72.307, 74.9274) (71.7674, 75.1509) (71.2048, 75.1509) knots 0 0 0 0 1 1 1 1 projected
  spline S221 degree 3 poles (73.3261, 73.0296) (73.3261, 73.5922) (73.1026, 74.1318) (72.7048, 74.5296) knots 0 0 0 0 1 1 1 1 projected
  spline S222 degree 3 poles (72.0166, 71.0698) (72.8093, 71.3981) (73.3261, 72.1716) (73.3261, 73.0296) knots 0 0 0 0 1 1 1 1 projected
  spline S223 degree 3 poles (69.7048, 71.5296) (70.3115, 70.9229) (71.2239, 70.7414) (72.0166, 71.0698) knots 0 0 0 0 1 1 1 1 projected
  spline S224 degree 3 poles (69.245, 73.8414) (68.9166, 73.0487) (69.0981, 72.1363) (69.7048, 71.5296) knots 0 0 0 0 1 1 1 1 projected
  spline S225 degree 3 poles (71.2048, 75.1509) (70.3468, 75.1509) (69.5733, 74.6341) (69.245, 73.8414) knots 0 0 0 0 1 1 1 1 projected
  spline S226 degree 3 poles (60.3068, 90.5796) (60.9135, 89.9729) (61.8259, 89.7914) (62.6186, 90.1198) knots 0 0 0 0 1 1 1 1 projected
  spline S227 degree 3 poles (59.847, 92.8914) (59.5186, 92.0987) (59.7001, 91.1863) (60.3068, 90.5796) knots 0 0 0 0 1 1 1 1 projected
  spline S228 degree 3 poles (62.6186, 90.1198) (63.4113, 90.4481) (63.9281, 91.2216) (63.9281, 92.0796) knots 0 0 0 0 1 1 1 1 projected
  spline S229 degree 3 poles (63.9281, 92.0796) (63.9281, 92.6422) (63.7046, 93.1818) (63.3068, 93.5796) knots 0 0 0 0 1 1 1 1 projected
  spline S230 degree 3 poles (63.3068, 93.5796) (62.909, 93.9774) (62.3694, 94.2009) (61.8068, 94.2009) knots 0 0 0 0 1 1 1 1 projected
  spline S231 degree 3 poles (78.897, 92.8914) (78.5686, 92.0987) (78.7501, 91.1863) (79.3568, 90.5796) knots 0 0 0 0 1 1 1 1 projected
  spline S232 degree 3 poles (79.3568, 90.5796) (79.9635, 89.9729) (80.8759, 89.7914) (81.6686, 90.1198) knots 0 0 0 0 1 1 1 1 projected
  spline S233 degree 3 poles (80.8568, 94.2009) (79.9988, 94.2009) (79.2253, 93.6841) (78.897, 92.8914) knots 0 0 0 0 1 1 1 1 projected
  spline S234 degree 3 poles (81.6686, 90.1198) (82.4613, 90.4481) (82.9781, 91.2216) (82.9781, 92.0796) knots 0 0 0 0 1 1 1 1 projected
  spline S235 degree 3 poles (82.9781, 92.0796) (82.9781, 93.2512) (82.0284, 94.2009) (80.8568, 94.2009) knots 0 0 0 0 1 1 1 1 projected
  spline S236 degree 3 poles (61.8068, 94.2009) (60.9488, 94.2009) (60.1753, 93.6841) (59.847, 92.8914) knots 0 0 0 0 1 1 1 1 projected
  spline S237 degree 3 poles (50.1726, 13.9198) (50.9653, 14.2481) (51.4821, 15.0216) (51.4821, 15.8796) knots 0 0 0 0 1 1 1 1 projected
  spline S238 degree 3 poles (50.8608, 17.3796) (50.463, 17.7774) (49.9234, 18.0009) (49.3608, 18.0009) knots 0 0 0 0 1 1 1 1 projected
  spline S239 degree 3 poles (49.3608, 18.0009) (48.5028, 18.0009) (47.7293, 17.4841) (47.401, 16.6914) knots 0 0 0 0 1 1 1 1 projected
  spline S240 degree 3 poles (47.8608, 14.3796) (48.4675, 13.7729) (49.3799, 13.5914) (50.1726, 13.9198) knots 0 0 0 0 1 1 1 1 projected
  spline S241 degree 3 poles (47.401, 16.6914) (47.0726, 15.8987) (47.2541, 14.9863) (47.8608, 14.3796) knots 0 0 0 0 1 1 1 1 projected
  spline S242 degree 3 poles (51.4821, 15.8796) (51.4821, 16.4422) (51.2586, 16.9818) (50.8608, 17.3796) knots 0 0 0 0 1 1 1 1 projected
  line L20 (51.7568, 67.0296) -> (51.7568, 82.0296) projected
  line L21 (57.7568, 67.0296) -> (51.7568, 67.0296) projected
  line L22 (57.7568, 82.0296) -> (57.7568, 67.0296) projected
  line L23 (51.7568, 82.0296) -> (57.7568, 82.0296) projected
  line L24 (27.7568, 67.0296) -> (27.7568, 82.0296) projected
  line L25 (33.7568, 67.0296) -> (27.7568, 67.0296) projected
  line L26 (33.7568, 82.0296) -> (33.7568, 67.0296) projected
  line L27 (27.7568, 82.0296) -> (33.7568, 82.0296) projected
  spline S243 degree 3 poles (40.1501, 92.0796) (40.1501, 92.6422) (39.9266, 93.1818) (39.5288, 93.5796) knots 0 0 0 0 1 1 1 1 projected
  spline S244 degree 3 poles (39.5288, 93.5796) (39.131, 93.9774) (38.5914, 94.2009) (38.0288, 94.2009) knots 0 0 0 0 1 1 1 1 projected
  spline S245 degree 3 poles (38.0288, 89.9583) (39.2004, 89.9583) (40.1501, 90.908) (40.1501, 92.0796) knots 0 0 0 0 1 1 1 1 projected
  spline S246 degree 3 poles (38.0288, 94.2009) (36.8572, 94.2009) (35.9075, 93.2512) (35.9075, 92.0796) knots 0 0 0 0 1 1 1 1 projected
  spline S247 degree 3 poles (35.9075, 92.0796) (35.9075, 90.908) (36.8572, 89.9583) (38.0288, 89.9583) knots 0 0 0 0 1 1 1 1 projected
  spline S248 degree 3 poles (44.8781, 73.0296) (44.8781, 73.5922) (44.6546, 74.1318) (44.2568, 74.5296) knots 0 0 0 0 1 1 1 1 projected
  spline S249 degree 3 poles (44.2568, 74.5296) (43.859, 74.9274) (43.3194, 75.1509) (42.7568, 75.1509) knots 0 0 0 0 1 1 1 1 projected
  spline S250 degree 3 poles (43.5686, 71.0698) (44.3613, 71.3981) (44.8781, 72.1716) (44.8781, 73.0296) knots 0 0 0 0 1 1 1 1 projected
  spline S251 degree 3 poles (42.7568, 75.1509) (41.8988, 75.1509) (41.1253, 74.6341) (40.797, 73.8414) knots 0 0 0 0 1 1 1 1 projected
  spline S252 degree 3 poles (40.797, 73.8414) (40.4686, 73.0487) (40.6501, 72.1363) (41.2568, 71.5296) knots 0 0 0 0 1 1 1 1 projected
  spline S253 degree 3 poles (41.2568, 71.5296) (41.8635, 70.9229) (42.7759, 70.7414) (43.5686, 71.0698) knots 0 0 0 0 1 1 1 1 projected
  spline S254 degree 3 poles (56.9808, 56.1009) (56.1228, 56.1009) (55.3493, 55.5841) (55.021, 54.7914) knots 0 0 0 0 1 1 1 1 projected
  spline S255 degree 3 poles (57.7926, 52.0198) (58.5853, 52.3481) (59.1021, 53.1216) (59.1021, 53.9796) knots 0 0 0 0 1 1 1 1 projected
  spline S256 degree 3 poles (55.021, 54.7914) (54.6926, 53.9987) (54.8741, 53.0863) (55.4808, 52.4796) knots 0 0 0 0 1 1 1 1 projected
  spline S257 degree 3 poles (55.4808, 52.4796) (56.0875, 51.8729) (56.9999, 51.6914) (57.7926, 52.0198) knots 0 0 0 0 1 1 1 1 projected
  spline S258 degree 3 poles (37.7661, 53.9796) (37.7661, 54.5422) (37.5426, 55.0818) (37.1448, 55.4796) knots 0 0 0 0 1 1 1 1 projected
  spline S259 degree 3 poles (37.1448, 55.4796) (36.747, 55.8774) (36.2074, 56.1009) (35.6448, 56.1009) knots 0 0 0 0 1 1 1 1 projected
  spline S260 degree 3 poles (36.4566, 52.0198) (37.2493, 52.3481) (37.7661, 53.1216) (37.7661, 53.9796) knots 0 0 0 0 1 1 1 1 projected
  spline S261 degree 3 poles (35.6448, 56.1009) (34.7868, 56.1009) (34.0133, 55.5841) (33.685, 54.7914) knots 0 0 0 0 1 1 1 1 projected
  spline S262 degree 3 poles (33.685, 54.7914) (33.3566, 53.9987) (33.5381, 53.0863) (34.1448, 52.4796) knots 0 0 0 0 1 1 1 1 projected
  spline S263 degree 3 poles (34.1448, 52.4796) (34.7515, 51.8729) (35.6639, 51.6914) (36.4566, 52.0198) knots 0 0 0 0 1 1 1 1 projected
  spline S264 degree 3 poles (59.1021, 53.9796) (59.1021, 55.1512) (58.1524, 56.1009) (56.9808, 56.1009) knots 0 0 0 0 1 1 1 1 projected
  spline S265 degree 3 poles (28.7374, 107.6258) (28.4092, 107.954) (27.9641, 108.1384) (27.5, 108.1384) knots 0 0 0 0 1 1 1 1 projected
  spline S266 degree 3 poles (29.25, 106.3884) (29.25, 106.8525) (29.0656, 107.2976) (28.7374, 107.6258) knots 0 0 0 0 1 1 1 1 projected
  spline S267 degree 3 poles (28.1697, 104.7716) (28.8236, 105.0425) (29.25, 105.6806) (29.25, 106.3884) knots 0 0 0 0 1 1 1 1 projected
  spline S268 degree 3 poles (26.2626, 105.151) (26.7631, 104.6505) (27.5158, 104.5007) (28.1697, 104.7716) knots 0 0 0 0 1 1 1 1 projected
  spline S269 degree 3 poles (25.8832, 107.0581) (25.6123, 106.4042) (25.7621, 105.6515) (26.2626, 105.151) knots 0 0 0 0 1 1 1 1 projected
  spline S270 degree 3 poles (27.5, 108.1384) (26.7922, 108.1384) (26.1541, 107.712) (25.8832, 107.0581) knots 0 0 0 0 1 1 1 1 projected
  spline S271 degree 3 poles (34.8588, 122.1384) (34.461, 122.5362) (33.9214, 122.7597) (33.3588, 122.7597) knots 0 0 0 0 1 1 1 1 projected
  spline S272 degree 3 poles (35.4801, 120.6384) (35.4801, 121.201) (35.2566, 121.7406) (34.8588, 122.1384) knots 0 0 0 0 1 1 1 1 projected
  spline S273 degree 3 poles (34.1706, 118.6786) (34.9633, 119.0069) (35.4801, 119.7804) (35.4801, 120.6384) knots 0 0 0 0 1 1 1 1 projected
  spline S274 degree 3 poles (31.8588, 119.1384) (32.4655, 118.5317) (33.3779, 118.3502) (34.1706, 118.6786) knots 0 0 0 0 1 1 1 1 projected
  spline S275 degree 3 poles (31.399, 121.4502) (31.0706, 120.6575) (31.2521, 119.7451) (31.8588, 119.1384) knots 0 0 0 0 1 1 1 1 projected
  spline S276 degree 3 poles (33.3588, 122.7597) (32.5008, 122.7597) (31.7273, 122.2429) (31.399, 121.4502) knots 0 0 0 0 1 1 1 1 projected
  spline S277 degree 3 poles (65.9072, 122.3516) (65.5094, 122.7494) (64.9698, 122.9729) (64.4072, 122.9729) knots 0 0 0 0 1 1 1 1 projected
  spline S278 degree 3 poles (66.5285, 120.8516) (66.5285, 121.4142) (66.305, 121.9538) (65.9072, 122.3516) knots 0 0 0 0 1 1 1 1 projected
  spline S279 degree 3 poles (65.219, 118.8918) (66.0117, 119.2201) (66.5285, 119.9936) (66.5285, 120.8516) knots 0 0 0 0 1 1 1 1 projected
  spline S280 degree 3 poles (62.9072, 119.3516) (63.5139, 118.7449) (64.4263, 118.5634) (65.219, 118.8918) knots 0 0 0 0 1 1 1 1 projected
  spline S281 degree 3 poles (62.4474, 121.6634) (62.119, 120.8707) (62.3005, 119.9583) (62.9072, 119.3516) knots 0 0 0 0 1 1 1 1 projected
  spline S282 degree 3 poles (64.4072, 122.9729) (63.5492, 122.9729) (62.7757, 122.4561) (62.4474, 121.6634) knots 0 0 0 0 1 1 1 1 projected
  spline S283 degree 3 poles (90.3441, 120.7364) (90.3441, 121.299) (90.1206, 121.8386) (89.7228, 122.2364) knots 0 0 0 0 1 1 1 1 projected
  spline S284 degree 3 poles (86.7228, 119.2364) (87.3295, 118.6297) (88.2419, 118.4482) (89.0346, 118.7766) knots 0 0 0 0 1 1 1 1 projected
  spline S285 degree 3 poles (86.263, 121.5482) (85.9346, 120.7555) (86.1161, 119.8431) (86.7228, 119.2364) knots 0 0 0 0 1 1 1 1 projected
  spline S286 degree 3 poles (88.2228, 122.8577) (87.3648, 122.8577) (86.5913, 122.3409) (86.263, 121.5482) knots 0 0 0 0 1 1 1 1 projected
  spline S287 degree 3 poles (89.7228, 122.2364) (89.325, 122.6342) (88.7854, 122.8577) (88.2228, 122.8577) knots 0 0 0 0 1 1 1 1 projected
  spline S288 degree 3 poles (28.7374, 45.4874) (28.4092, 45.8156) (27.9641, 46) (27.5, 46) knots 0 0 0 0 1 1 1 1 projected
  spline S289 degree 3 poles (29.25, 44.25) (29.25, 44.7141) (29.0656, 45.1592) (28.7374, 45.4874) knots 0 0 0 0 1 1 1 1 projected
  spline S290 degree 3 poles (28.1697, 42.6332) (28.8236, 42.9041) (29.25, 43.5422) (29.25, 44.25) knots 0 0 0 0 1 1 1 1 projected
  spline S291 degree 3 poles (26.2626, 43.0126) (26.7631, 42.5121) (27.5158, 42.3623) (28.1697, 42.6332) knots 0 0 0 0 1 1 1 1 projected
  spline S292 degree 3 poles (42.5921, 34.9296) (42.5921, 35.4922) (42.3686, 36.0318) (41.9708, 36.4296) knots 0 0 0 0 1 1 1 1 projected
  spline S293 degree 3 poles (41.2826, 32.9698) (42.0753, 33.2981) (42.5921, 34.0716) (42.5921, 34.9296) knots 0 0 0 0 1 1 1 1 projected
  spline S294 degree 3 poles (41.9708, 36.4296) (41.573, 36.8274) (41.0334, 37.0509) (40.4708, 37.0509) knots 0 0 0 0 1 1 1 1 projected
  spline S295 degree 3 poles (38.9708, 33.4296) (39.5775, 32.8229) (40.4899, 32.6414) (41.2826, 32.9698) knots 0 0 0 0 1 1 1 1 projected
  spline S296 degree 3 poles (40.4708, 37.0509) (39.6128, 37.0509) (38.8393, 36.5341) (38.511, 35.7414) knots 0 0 0 0 1 1 1 1 projected
  spline S297 degree 3 poles (38.511, 35.7414) (38.1826, 34.9487) (38.3641, 34.0363) (38.9708, 33.4296) knots 0 0 0 0 1 1 1 1 projected
  line L28 (101.6246, 9.8046) -> (101.6246, 24.8046) projected
  line L29 (107.6246, 9.8046) -> (101.6246, 9.8046) projected
  line L30 (107.6246, 24.8046) -> (107.6246, 9.8046) projected
  spline S298 degree 3 poles (68.1328, 36.4296) (67.735, 36.8274) (67.1954, 37.0509) (66.6328, 37.0509) knots 0 0 0 0 1 1 1 1 projected
  spline S299 degree 3 poles (73.2368, 18.0009) (72.3788, 18.0009) (71.6053, 17.4841) (71.277, 16.6914) knots 0 0 0 0 1 1 1 1 projected
  spline S300 degree 3 poles (71.7368, 14.3796) (72.3435, 13.7729) (73.2559, 13.5914) (74.0486, 13.9198) knots 0 0 0 0 1 1 1 1 projected
  spline S301 degree 3 poles (64.673, 35.7414) (64.3446, 34.9487) (64.5261, 34.0363) (65.1328, 33.4296) knots 0 0 0 0 1 1 1 1 projected
  spline S302 degree 3 poles (65.1328, 33.4296) (65.7395, 32.8229) (66.6519, 32.6414) (67.4446, 32.9698) knots 0 0 0 0 1 1 1 1 projected
  spline S303 degree 3 poles (66.6328, 37.0509) (65.7748, 37.0509) (65.0013, 36.5341) (64.673, 35.7414) knots 0 0 0 0 1 1 1 1 projected
  spline S304 degree 3 poles (74.0486, 13.9198) (74.8413, 14.2481) (75.3581, 15.0216) (75.3581, 15.8796) knots 0 0 0 0 1 1 1 1 projected
  spline S305 degree 3 poles (74.7368, 17.3796) (74.339, 17.7774) (73.7994, 18.0009) (73.2368, 18.0009) knots 0 0 0 0 1 1 1 1 projected
  spline S306 degree 3 poles (75.3581, 15.8796) (75.3581, 16.4422) (75.1346, 16.9818) (74.7368, 17.3796) knots 0 0 0 0 1 1 1 1 projected
  spline S307 degree 3 poles (67.4446, 32.9698) (68.2373, 33.2981) (68.7541, 34.0716) (68.7541, 34.9296) knots 0 0 0 0 1 1 1 1 projected
  spline S308 degree 3 poles (68.7541, 34.9296) (68.7541, 35.4922) (68.5306, 36.0318) (68.1328, 36.4296) knots 0 0 0 0 1 1 1 1 projected
  spline S309 degree 3 poles (83.5615, 34.9296) (83.5615, 33.758) (84.5112, 32.8083) (85.6828, 32.8083) knots 0 0 0 0 1 1 1 1 projected
  spline S310 degree 3 poles (85.6828, 37.0509) (84.5112, 37.0509) (83.5615, 36.1012) (83.5615, 34.9296) knots 0 0 0 0 1 1 1 1 projected
  spline S311 degree 3 poles (85.6828, 32.8083) (86.8544, 32.8083) (87.8041, 33.758) (87.8041, 34.9296) knots 0 0 0 0 1 1 1 1 projected
  spline S312 degree 3 poles (87.1828, 36.4296) (86.785, 36.8274) (86.2454, 37.0509) (85.6828, 37.0509) knots 0 0 0 0 1 1 1 1 projected
  spline S313 degree 3 poles (87.8041, 34.9296) (87.8041, 35.4922) (87.5806, 36.0318) (87.1828, 36.4296) knots 0 0 0 0 1 1 1 1 projected
  spline S314 degree 3 poles (74.5308, 52.4796) (75.1375, 51.8729) (76.0499, 51.6914) (76.8426, 52.0198) knots 0 0 0 0 1 1 1 1 projected
  spline S315 degree 3 poles (74.071, 54.7914) (73.7426, 53.9987) (73.9241, 53.0863) (74.5308, 52.4796) knots 0 0 0 0 1 1 1 1 projected
  spline S316 degree 3 poles (76.8426, 52.0198) (77.6353, 52.3481) (78.1521, 53.1216) (78.1521, 53.9796) knots 0 0 0 0 1 1 1 1 projected
  spline S317 degree 3 poles (76.0308, 56.1009) (75.1728, 56.1009) (74.3993, 55.5841) (74.071, 54.7914) knots 0 0 0 0 1 1 1 1 projected
  spline S318 degree 3 poles (78.1521, 53.9796) (78.1521, 54.5422) (77.9286, 55.0818) (77.5308, 55.4796) knots 0 0 0 0 1 1 1 1 projected
  spline S319 degree 3 poles (77.5308, 55.4796) (77.133, 55.8774) (76.5934, 56.1009) (76.0308, 56.1009) knots 0 0 0 0 1 1 1 1 projected
  spline S320 degree 3 poles (92.9595, 53.9796) (92.9595, 52.808) (93.9092, 51.8583) (95.0808, 51.8583) knots 0 0 0 0 1 1 1 1 projected
  spline S321 degree 3 poles (95.0808, 56.1009) (93.9092, 56.1009) (92.9595, 55.1512) (92.9595, 53.9796) knots 0 0 0 0 1 1 1 1 projected
  spline S322 degree 3 poles (96.5808, 55.4796) (96.183, 55.8774) (95.6434, 56.1009) (95.0808, 56.1009) knots 0 0 0 0 1 1 1 1 projected
  spline S323 degree 3 poles (97.2021, 53.9796) (97.2021, 54.5422) (96.9786, 55.0818) (96.5808, 55.4796) knots 0 0 0 0 1 1 1 1 projected
  spline S324 degree 3 poles (95.0808, 51.8583) (96.2524, 51.8583) (97.2021, 52.808) (97.2021, 53.9796) knots 0 0 0 0 1 1 1 1 projected
  spline S325 degree 3 poles (71.277, 16.6914) (70.9486, 15.8987) (71.1301, 14.9863) (71.7368, 14.3796) knots 0 0 0 0 1 1 1 1 projected
  spline S326 degree 3 poles (294.5601, 15.8796) (294.5601, 16.4422) (294.3366, 16.9818) (293.9388, 17.3796) knots 0 0 0 0 1 1 1 1 projected
  spline S327 degree 3 poles (293.9388, 17.3796) (293.541, 17.7774) (293.0014, 18.0009) (292.4388, 18.0009) knots 0 0 0 0 1 1 1 1 projected
  spline S328 degree 3 poles (292.4388, 13.7583) (293.6104, 13.7583) (294.5601, 14.708) (294.5601, 15.8796) knots 0 0 0 0 1 1 1 1 projected
  spline S329 degree 3 poles (294.4468, 36.4296) (294.049, 36.8274) (293.5094, 37.0509) (292.9468, 37.0509) knots 0 0 0 0 1 1 1 1 projected
  spline S330 degree 3 poles (290.987, 35.7414) (290.6586, 34.9487) (290.8401, 34.0363) (291.4468, 33.4296) knots 0 0 0 0 1 1 1 1 projected
  spline S331 degree 3 poles (292.4388, 18.0009) (291.2672, 18.0009) (290.3175, 17.0512) (290.3175, 15.8796) knots 0 0 0 0 1 1 1 1 projected
  spline S332 degree 3 poles (290.3175, 15.8796) (290.3175, 14.708) (291.2672, 13.7583) (292.4388, 13.7583) knots 0 0 0 0 1 1 1 1 projected
  line L31 (283.9468, 43.9296) -> (283.9468, 28.9296) projected
  spline S333 degree 3 poles (270.6841, 15.8796) (270.6841, 16.4422) (270.4606, 16.9818) (270.0628, 17.3796) knots 0 0 0 0 1 1 1 1 projected
  spline S334 degree 3 poles (269.3746, 13.9198) (270.1673, 14.2481) (270.6841, 15.0216) (270.6841, 15.8796) knots 0 0 0 0 1 1 1 1 projected
  spline S335 degree 3 poles (270.0628, 17.3796) (269.665, 17.7774) (269.1254, 18.0009) (268.5628, 18.0009) knots 0 0 0 0 1 1 1 1 projected
  spline S336 degree 3 poles (267.0628, 14.3796) (267.6695, 13.7729) (268.5819, 13.5914) (269.3746, 13.9198) knots 0 0 0 0 1 1 1 1 projected
  spline S337 degree 3 poles (268.5628, 18.0009) (267.7048, 18.0009) (266.9313, 17.4841) (266.603, 16.6914) knots 0 0 0 0 1 1 1 1 projected
  spline S338 degree 3 poles (308.6708, 64.8776) (308.273, 65.2754) (307.7334, 65.4989) (307.1708, 65.4989) knots 0 0 0 0 1 1 1 1 projected
  spline S339 degree 3 poles (309.2921, 63.3776) (309.2921, 63.9402) (309.0686, 64.4798) (308.6708, 64.8776) knots 0 0 0 0 1 1 1 1 projected
  spline S340 degree 3 poles (307.9826, 61.4178) (308.7753, 61.7461) (309.2921, 62.5196) (309.2921, 63.3776) knots 0 0 0 0 1 1 1 1 projected
  spline S341 degree 3 poles (305.6708, 61.8776) (306.2775, 61.2709) (307.1899, 61.0894) (307.9826, 61.4178) knots 0 0 0 0 1 1 1 1 projected
  spline S342 degree 3 poles (305.211, 64.1894) (304.8826, 63.3967) (305.0641, 62.4843) (305.6708, 61.8776) knots 0 0 0 0 1 1 1 1 projected
  spline S343 degree 3 poles (307.1708, 65.4989) (306.3128, 65.4989) (305.5393, 64.9821) (305.211, 64.1894) knots 0 0 0 0 1 1 1 1 projected
  spline S344 degree 3 poles (282.2548, 74.5296) (281.857, 74.9274) (281.3174, 75.1509) (280.7548, 75.1509) knots 0 0 0 0 1 1 1 1 projected
  spline S345 degree 3 poles (282.8761, 73.0296) (282.8761, 73.5922) (282.6526, 74.1318) (282.2548, 74.5296) knots 0 0 0 0 1 1 1 1 projected
  spline S346 degree 3 poles (281.5666, 71.0698) (282.3593, 71.3981) (282.8761, 72.1716) (282.8761, 73.0296) knots 0 0 0 0 1 1 1 1 projected
  spline S347 degree 3 poles (279.2548, 71.5296) (279.8615, 70.9229) (280.7739, 70.7414) (281.5666, 71.0698) knots 0 0 0 0 1 1 1 1 projected
  spline S348 degree 3 poles (278.795, 73.8414) (278.4666, 73.0487) (278.6481, 72.1363) (279.2548, 71.5296) knots 0 0 0 0 1 1 1 1 projected
  spline S349 degree 3 poles (280.7548, 75.1509) (279.8968, 75.1509) (279.1233, 74.6341) (278.795, 73.8414) knots 0 0 0 0 1 1 1 1 projected
  spline S350 degree 3 poles (263.2048, 74.5296) (262.807, 74.9274) (262.2674, 75.1509) (261.7048, 75.1509) knots 0 0 0 0 1 1 1 1 projected
  spline S351 degree 3 poles (263.8261, 73.0296) (263.8261, 73.5922) (263.6026, 74.1318) (263.2048, 74.5296) knots 0 0 0 0 1 1 1 1 projected
  spline S352 degree 3 poles (262.5166, 71.0698) (263.3093, 71.3981) (263.8261, 72.1716) (263.8261, 73.0296) knots 0 0 0 0 1 1 1 1 projected
  spline S353 degree 3 poles (260.2048, 71.5296) (260.8115, 70.9229) (261.7239, 70.7414) (262.5166, 71.0698) knots 0 0 0 0 1 1 1 1 projected
  spline S354 degree 3 poles (259.745, 73.8414) (259.4166, 73.0487) (259.5981, 72.1363) (260.2048, 71.5296) knots 0 0 0 0 1 1 1 1 projected
  spline S355 degree 3 poles (261.7048, 75.1509) (260.8468, 75.1509) (260.0733, 74.6341) (259.745, 73.8414) knots 0 0 0 0 1 1 1 1 projected
  spline S356 degree 3 poles (265.2848, 52.4796) (265.8915, 51.8729) (266.8039, 51.6914) (267.5966, 52.0198) knots 0 0 0 0 1 1 1 1 projected
  spline S357 degree 3 poles (267.5966, 52.0198) (268.3893, 52.3481) (268.9061, 53.1216) (268.9061, 53.9796) knots 0 0 0 0 1 1 1 1 projected
  spline S358 degree 3 poles (264.825, 54.7914) (264.4966, 53.9987) (264.6781, 53.0863) (265.2848, 52.4796) knots 0 0 0 0 1 1 1 1 projected
  spline S359 degree 3 poles (266.7848, 56.1009) (265.9268, 56.1009) (265.1533, 55.5841) (264.825, 54.7914) knots 0 0 0 0 1 1 1 1 projected
  spline S360 degree 3 poles (268.2848, 55.4796) (267.887, 55.8774) (267.3474, 56.1009) (266.7848, 56.1009) knots 0 0 0 0 1 1 1 1 projected
  spline S361 degree 3 poles (268.9061, 53.9796) (268.9061, 54.5422) (268.6826, 55.0818) (268.2848, 55.4796) knots 0 0 0 0 1 1 1 1 projected
  spline S362 degree 3 poles (283.7135, 53.9796) (283.7135, 52.808) (284.6632, 51.8583) (285.8348, 51.8583) knots 0 0 0 0 1 1 1 1 projected
  spline S363 degree 3 poles (285.8348, 51.8583) (287.0064, 51.8583) (287.9561, 52.808) (287.9561, 53.9796) knots 0 0 0 0 1 1 1 1 projected
  spline S364 degree 3 poles (285.8348, 56.1009) (284.6632, 56.1009) (283.7135, 55.1512) (283.7135, 53.9796) knots 0 0 0 0 1 1 1 1 projected
  spline S365 degree 3 poles (287.3348, 55.4796) (286.937, 55.8774) (286.3974, 56.1009) (285.8348, 56.1009) knots 0 0 0 0 1 1 1 1 projected
  spline S366 degree 3 poles (287.9561, 53.9796) (287.9561, 54.5422) (287.7326, 55.0818) (287.3348, 55.4796) knots 0 0 0 0 1 1 1 1 projected
  spline S367 degree 3 poles (255.6328, 33.4296) (256.2395, 32.8229) (257.1519, 32.6414) (257.9446, 32.9698) knots 0 0 0 0 1 1 1 1 projected
  spline S368 degree 3 poles (262.031, 121.5482) (261.7026, 120.7555) (261.8841, 119.8431) (262.4908, 119.2364) knots 0 0 0 0 1 1 1 1 projected